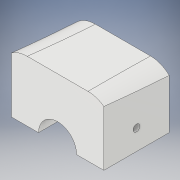
# Autodesk Inventor part: AA008
Saved by Autodesk Inventor 2017 SP1 (Build 210196100, 196)
## iProperties
Created: 2017-09-28
Part Number: AA008
Material: ABS Plastic
Document SubType Name: Modeling
Designer: Zach
Density: 1.06 g/cm^3
Appearance: CR White
Author: Zach
Autodesk Inventor part; units mm, degrees
ref_plane "YZ Plane" through (0, 0, 0) normal (1, 0, 0) x (0, 1, 0)
ref_plane "XZ Plane" through (0, 0, 0) normal (0, 1, 0) x (-1, 0, 0)
ref_plane "XY Plane" through (0, 0, 0) normal (0, 0, 1) x (1, 0, 0)
sketch "Sketch1" plane through (0, 0, 0) normal (0, 0, 1) x (1, 0, 0)
  line L0 (0, 0) -> (80, 0)
  line L1 (80, 0) -> (80, 82.6)
  line L2 (80, 82.6) -> (0, 82.6)
  line L3 (0, 82.6) -> (0, 0)
  dimension "d0" = 80
  dimension "d1" = 82.6
  constraints: 8 end point, 2 parallel, 1 horizontal, 1 perpendicular
  measures "d0" distance of L2.end L1.end
  measures "d1" distance of L1.end L0.end
extrude "Extrusion1" add sketch "Sketch1" along normal blind 162.5
sketch "Sketch2" plane through (0, 82.6, 0) normal (0, 1, 0) x (1, 0, 0)
  line L0 (0, -162.5) -> (80, -162.5) projected
  line L1 (-12.5, -162.5) -> (0, -162.5)
  line L2 (80, -162.5) -> (92.5, -162.5)
  line L3 (0, 0) -> (80, 0) projected
  line L4 (0, 0) -> (0, -162.5) projected
  line L5 (80, 0) -> (80, -162.5) projected
  arc A0 (-12.5, -162.5) -> (0, 0) centre (-1199.9534, 10.5733) ccw
  arc A1 (80, 0) -> (92.5, -162.5) centre (1279.9534, 10.5733) ccw
  dimension "d4" = 12.5
  dimension "d5" = 12.5
  dimension "d19" = 1200
  dimension "d20" = 1200
  constraints: 4 end point, 4 point on circle, 2 centre point, 1 collinear, 1 parallel
  measures "d4" distance of L1.start L0.start
  measures "d5" distance of L0.end L2.end
  measures "d19" radius of A0
  measures "d20" radius of A1
extrude "Extrusion2" add sketch "Sketch2" against normal blind 82.6 contours L1 A0 L4 | L5 A1 L2
sketch "Sketch4" plane through (0, 0, 0) normal (0, 0, -1) x (-1, 0, 0)
  circle A0 centre (-17.4, 59.41) radius 2.5
  circle A1 centre (-62.6, 59.41) radius 2.5
  circle A2 centre (-62.6, 23.19) radius 2.5
  circle A3 centre (-17.4, 23.19) radius 2.5
  line L0 (-80, 82.6) -> (0, 82.6) projected
  line L1 (-17.4, 23.19) -> (-62.6, 23.19) construction
  line L2 (-62.6, 23.19) -> (-62.6, 59.41) construction
  line L3 (-80, 0) -> (-80, 82.6) projected
  point P0 (0, 0)
  point P1 (-60.8187, 82.6)
  point P2 (-19.1813, 82.6)
  point P3 (-40, 23.19)
  point P4 (-40, 82.6)
  dimension "d10" = 5
  dimension "d11" = 5
  dimension "d12" = 5
  dimension "d13" = 5
  dimension "d14" = 23.19
  dimension "d15" = 45.2
  dimension "d16" = 36.22
  constraints: 4 centre point, 4 end point, 3 vertical alignment, 2 horizontal alignment, 2 midpoint, 1 horizontal, 1 perpendicular
  measures "d10" diameter of A0
  measures "d11" diameter of A1
  measures "d12" diameter of A2
  measures "d13" diameter of A3
  measures "d14" distance from line of L0 A0.centre
  measures "d15" distance of L2.end A0.centre
  measures "d16" distance of L2.end L1.end
extrude "Extrusion3" cut sketch "Sketch4" against normal blind 25
sketch "Sketch5" plane through (0, 0, 0) normal (0, 0, -1) x (-1, 0, 0)
  line L0 (12.5, 0) -> (-92.5, 0)
  line L1 (-92.5, 0) -> (-92.5, 41.3)
  line L2 (-92.5, 41.3) -> (12.5, 41.3)
  line L3 (12.5, 41.3) -> (12.5, 0)
  point P0 (0, 0)
  point P1 (12.5, 20)
  point P2 (-92.5, 20)
  dimension "d22" = 41.3
  constraints: 8 end point, 2 parallel, 2 point on line, 1 horizontal, 1 horizontal alignment, 1 perpendicular
  measures "d22" distance of L0.end L1.end
extrude "Extrusion4" cut sketch "Sketch5" against normal through all
sketch "Sketch6" plane through (0, 41.3, 0) normal (0, -1, 0) x (1, 0, 0)
  line L0 (75, 15) -> (5, 15)
  line L1 (5, 15) -> (5, 65)
  line L2 (5, 65) -> (75, 65)
  line L3 (75, 65) -> (75, 15)
  line L4 (80, 0) -> (0, 0) projected
  point P0 (40, 15)
  point P1 (40, 0)
  dimension "d25" = 70
  dimension "d26" = 50
  dimension "d27" = 15
  constraints: 8 end point, 2 midpoint, 2 parallel, 1 horizontal, 1 perpendicular, 1 vertical alignment
  measures "d25" distance of L1.end L2.end
  measures "d26" distance of L0.end L1.end
  measures "d27" distance between parallel lines of L4 L0
extrude "Extrusion5" cut sketch "Sketch6" against normal blind 32.5
sketch "Sketch8" plane through (0, 0, 0) normal (1, 0, 0) x (0, 1, 0)
  line L0 (82.6, 162.5) -> (93.8, 162.5)
  line L1 (41.3, 162.5) -> (41.3, 0) projected
  line L2 (82.6, 0) -> (41.3, 0) projected
  arc A0 (93.8, 162.5) -> (82.6, 0) centre (2580.9593, -90.5586) ccw
  line L3 (82.6, 162.5) -> (41.3, 162.5) projected
  line L4 (82.6, 162.5) -> (82.6, 0)
  point P0 (0, 0)
  dimension "d32" = 2500
  dimension "d38" = 11.2
  constraints: 4 end point, 2 point on circle, 1 centre point, 1 horizontal, 1 perpendicular
  measures "d32" radius of A0
  measures "d38" distance of L0.start L0.end
extrude "Extrusion6" add sketch "Sketch8" along normal blind 93 and the other way blind 13 contours L0 A0 L4
sketch "Sketch13" plane through (-13, 82.6, 0) normal (0, -1, 0) x (1, 0, 0)
  arc A0 (13, 0) -> (0.5, 162.5) centre (-1186.9534, -10.5733) ccw projected
  line L0 (0, 162.5) -> (0.5, 162.5) projected
  line L1 (0, 0) -> (0, 162.5) projected
  line L2 (13, 0) -> (0, 0) projected
  arc A1 (105.5, 162.5) -> (93, 0) centre (1292.9534, -10.5733) ccw projected
  line L3 (106, 0) -> (93, 0) projected
  line L4 (106, 162.5) -> (106, 0) projected
  line L5 (105.5, 162.5) -> (106, 162.5) projected
  point P0 (13, 0)
extrude "Extrusion9" cut sketch "Sketch13" against normal through all
fillet "Fillet4" radius 20 2 edges at (-3.5176, 86.9111, 81.8462) (83.5176, 86.9111, 81.8462)
sketch "Sketch34" plane through (0, 41.3, 0) normal (0, -1, 0) x (1, 0, 0)
  line L0 (75, 65) -> (75, 15) projected
  line L1 (75, 15) -> (5, 15) projected
  line L2 (5, 15) -> (5, 65) projected
  line L3 (5, 65) -> (75, 65) projected
  arc A0 (0, 0) -> (-12.5, 162.5) centre (-1199.9534, -10.5733) ccw projected
  line L4 (80, 0) -> (0, 0) projected
  arc A1 (92.5, 162.5) -> (80, 0) centre (1279.9534, -10.5733) ccw projected
  line L5 (-12.5, 162.5) -> (92.5, 162.5) projected
  point P0 (0, 0)
extrude "Extrusion24" cut sketch "Sketch34" against normal through all
sketch "Sketch35" plane through (0, 73.8, 0) normal (0, -1, 0) x (1, 0, 0)
  line L0 (75, 15) -> (5, 15) projected
  line L1 (75, 65) -> (75, 15) projected
  line L2 (5, 65) -> (75, 65) projected
  line L3 (5, 15) -> (5, 65) projected
  point P0 (0, 0)
extrude "Extrusion25" add sketch "Sketch35" along normal blind 32.5
sketch "Sketch36" plane through (0, 41.3, 0) normal (0, -1, 0) x (1, 0, 0)
  line L0 (10, 15) -> (70, 15)
  line L1 (70, 15) -> (70, 23)
  line L2 (70, 23) -> (10, 23)
  line L3 (10, 23) -> (10, 15)
  line L4 (5, 15) -> (75, 15) projected
  point P0 (0, 0)
  point P1 (40, 23)
  point P2 (40, 15)
  point P3 (40, 15)
  dimension "d112" = 8
  dimension "d113" = 60
  constraints: 8 end point, 3 midpoint, 2 parallel, 2 vertical alignment, 1 horizontal, 1 perpendicular, 1 point on line
  measures "d112" distance between parallel lines of L2 L0
  measures "d113" distance of L1.end L2.end
extrude "Extrusion26" cut sketch "Sketch36" against normal blind 32.5
sketch "Sketch37" plane through (5, 41.3, 65) normal (-1, 0, 0) x (0, 0, 1)
  circle A0 centre (-25, 15) radius 2.5
  line L0 (0, 0) -> (-50, 0) projected
  point P0 (-65, -41.3)
  point P1 (-25, 0)
  dimension "d116" = 5
  dimension "d117" = 15
  constraints: 1 centre point, 1 midpoint, 1 vertical alignment
  measures "d116" diameter of A0
  measures "d117" distance from line of L0 A0.centre
extrude "Extrusion27" cut sketch "Sketch37" against normal through all
sketch "Sketch38" plane through (0, 41.3, 0) normal (0, -1, 0) x (1, 0, 0)
  line L0 (75, 15) -> (5, 15)
  line L1 (5, 15) -> (5, 65)
  line L2 (5, 65) -> (75, 65)
  line L3 (75, 65) -> (75, 15)
  line L4 (75, 65) -> (5, 65) projected
  line L5 (75, 15) -> (75, 65) projected
  line L6 (74, 16) -> (6, 16)
  line L7 (6, 16) -> (6, 64)
  line L8 (6, 64) -> (74, 64)
  line L9 (74, 64) -> (74, 16)
  point P0 (0, 0)
  dimension "d120" = 1
  constraints: 16 end point, 4 parallel, 2 perpendicular, 1 horizontal, 3 other
  measures "d120" distance between parallel lines of L3 L9
extrude "Extrusion28" cut sketch "Sketch38" against normal through all
sketch "Sketch39" plane through (6, 41.3, 64) normal (0, 0, 1) x (1, 0, 0)
  line L0 (68, 0) -> (0, 0) projected
  line L1 (4, 0) -> (64, 0) projected
  circle A0 centre (34, 0) radius 14
  point P0 (-6, -41.3)
  dimension "d123" = 28
  constraints: 1 centre point, 1 midpoint
  measures "d123" diameter of A0
extrude "Extrusion29" cut sketch "Sketch39" against normal blind 25
equation "\"d5\" = d4"
body "Solid1"
